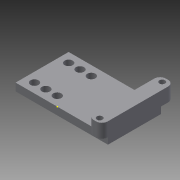
# Autodesk Inventor part: CartServoMount
Saved by Autodesk Inventor 2015 (Build 190159000, 159)
## iProperties
Created: 2016-03-27
Part Number: CartServoMount
Material: Generic
Document SubType Name: Modeling
Designer: Hatch
Density: 1 g/cm^3
Appearance: Default
Author: Hatch
Autodesk Inventor part; units mm, degrees
ref_plane "YZ Plane" through (0, 0, 0) normal (1, 0, 0) x (0, 1, 0)
ref_plane "XZ Plane" through (0, 0, 0) normal (0, 1, 0) x (-1, 0, 0)
ref_plane "XY Plane" through (0, 0, 0) normal (0, 0, 1) x (1, 0, 0)
sketch "Sketch2" plane through (0, 0, 0) normal (0, 1, 0) x (-1, 0, 0)
  line L0 (0, 0) -> (0, -28)
  line L1 (0, -28) -> (22, -28)
  line L2 (22, -28) -> (22, 0)
  line L3 (22, 0) -> (0, 0)
  dimension "d0" = 28
  dimension "d1" = 22
  constraints: 8 end point, 2 parallel, 1 perpendicular, 1 vertical
  measures "d0" distance of L0.start L0.end
  measures "d1" distance of L1.end L0.end
extrude "Extrusion1" add sketch "Sketch2" along normal blind 4
sketch "Sketch3" plane through (0, 4, 0) normal (0, 1, 0) x (1, 0, 0)
  line L0 (0, 0) -> (0, 5)
  line L1 (0, 0) -> (0, 28) projected
  line L2 (0, 5) -> (-5, 5)
  circle A0 centre (-5, 5) radius 2.125
  dimension "d4" = 5
  dimension "d5" = 5
  dimension "d6" = 4.25
  constraints: 4 end point, 1 centre point, 1 coincident, 1 perpendicular, 1 point on line
  measures "d4" distance of L0.start L0.end
  measures "d5" distance of L0.end L2.end
  measures "d6" diameter of A0
extrude "Extrusion2" cut sketch "Sketch3" against normal through all
pattern_linear "Rectangular Pattern1" count 2 spacing 18 along (0, 0, -1) count 3 spacing 6 along (-1, 0, 0) of "Extrusion2"
sketch "Sketch4" plane through (0, 4, 0) normal (0, 1, 0) x (1, 0, 0)
  point P0 (0, 0)
sketch "Sketch5" plane through (0, 0, 0) normal (1, 0, 0) x (0, 0, -1)
  line L0 (0, 4) -> (28, 4)
  line L1 (28, 4) -> (28, 0)
  line L2 (28, 0) -> (0, 0)
  line L3 (0, 0) -> (0, 4)
  line L4 (0, 4) -> (28, 4) projected
  constraints: 8 end point, 3 equal length, 1 perpendicular
extrude "Extrusion3" add sketch "Sketch5" along normal blind 21.25
sketch "Sketch6" plane through (0, 0, 0) normal (0, -1, 0) x (1, 0, 0)
  line L0 (21.25, 0) -> (26.75, 0)
  line L1 (26.75, 0) -> (26.75, -28)
  line L2 (26.75, -28) -> (21.25, -28)
  line L3 (21.25, -28) -> (21.25, 0)
  point P0 (0, 0)
  dimension "d17" = 5.5
  constraints: 8 end point, 2 parallel, 1 horizontal, 1 perpendicular
  measures "d17" distance of L1.end L2.end
extrude "Extrusion4" add sketch "Sketch6" against normal blind 12.5
sketch "Sketch7" plane through (26.75, 0, 0) normal (1, 0, 0) x (0, 0, -1)
  line L0 (0, 4) -> (0, 12.5) projected
  line L1 (28, 12.5) -> (0, 12.5)
  line L2 (0, 12.5) -> (0, 5.25)
  line L3 (0, 5.25) -> (28, 5.25)
  line L4 (28, 5.25) -> (28, 12.5)
  point P0 (0, 0)
  dimension "d20" = 7.25
  constraints: 8 end point, 2 parallel, 1 horizontal, 1 perpendicular, 1 point on line
  measures "d20" distance of L2.end L1.end
extrude "Extrusion5" add sketch "Sketch7" along normal blind 1.8
sketch "Sketch8" plane through (-22, 0, 0) normal (0, 0, 1) x (1, 0, 0)
  line L0 (50.55, 5.25) -> (43.25, 5.25)
  line L1 (43.25, 5.25) -> (43.25, 12.5)
  line L2 (43.25, 12.5) -> (50.55, 12.5)
  line L3 (50.55, 12.5) -> (50.55, 5.25)
  point P0 (22, 0)
  constraints: 8 end point, 2 parallel, 1 horizontal, 1 perpendicular
extrude "Extrusion6" add sketch "Sketch8" along normal blind 5
fillet "Fillet1" radius 3 1 edges at (21.25, 8.875, 5)
fillet "Fillet2" radius 3 1 edges at (28.55, 8.875, 5)
sketch "Sketch9" plane through (-22, 0, -28) normal (0, 0, -1) x (-1, 0, 0)
  line L0 (-43.25, 12.5) -> (-50.55, 12.5)
  line L1 (-50.55, 12.5) -> (-50.55, 5.25)
  line L2 (-50.55, 5.25) -> (-43.25, 5.25)
  line L3 (-43.25, 5.25) -> (-43.25, 12.5)
  point P0 (-22, 0)
  constraints: 8 end point, 2 parallel, 1 horizontal, 1 perpendicular
extrude "Extrusion7" add sketch "Sketch9" along normal blind 5
fillet "Fillet3" radius 3 1 edges at (28.55, 8.875, -33)
fillet "Fillet4" radius 3 1 edges at (21.25, 8.875, -33)
sketch "Sketch10" plane through (0, 12.5, 0) normal (0, 1, 0) x (1, 0, 0)
  line L0 (21.25, 28) -> (28.55, 28)
  line L1 (28.55, 30) -> (28.55, -2) projected
  line L2 (21.25, 28) -> (26.75, 28) projected
  line L3 (21.25, 0) -> (28.55, 0)
  line L4 (26.75, 0) -> (21.25, 0) projected
  line L5 (25.55, 33) -> (24.25, 33) projected
  line L6 (24.9, 33) -> (24.9, 28)
  line L7 (24.25, -5) -> (25.55, -5) projected
  line L8 (24.9, -5) -> (24.9, 0)
  circle A0 centre (24.9, 30.5) radius 1.5
  circle A1 centre (24.9, -2.5) radius 1.5
  point P0 (0, 0)
  dimension "d31" = 3
  dimension "d32" = 3
  constraints: 8 end point, 5 point on line, 4 midpoint, 2 centre point, 2 collinear, 1 perpendicular
  measures "d31" diameter of A0
  measures "d32" diameter of A1
extrude "Extrusion8" cut sketch "Sketch10" against normal through all
body "Solid1"
